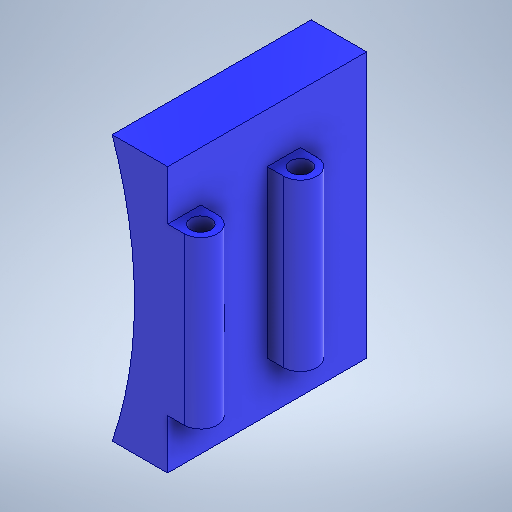
# Autodesk Inventor part: hand2_13
Saved by Autodesk Inventor 2025.1 (Build 291241000, 241)
## iProperties
Created: 2025-02-05
Part Number: hand2_13
Material: ABS プラスチック
Document SubType Name: Modeling
Designer: ryogo
Density: 1.06 g/cm^3
Appearance: 青 - 壁塗料 - 光沢
Author: ryogo
Autodesk Inventor part; units mm, degrees
ref_plane "YZ Plane" through (0, 0, 0) normal (1, 0, 0) x (0, 1, 0)
ref_plane "XZ Plane" through (0, 0, 0) normal (0, 1, 0) x (-1, 0, 0)
sketch "スケッチ1" plane through (0, 0, 0) normal (0, 1, 0) x (-1, 0, 0)
  line L0 (0, 0) -> (0, -30)
  circle A0 centre (0, 0) radius 3.05
  circle A1 centre (0, -30) radius 3.05
  circle A2 centre (0, 0) radius 5
  circle A3 centre (0, -30) radius 5
  line L1 (5, 0) -> (5, -30)
  line L2 (0, -5) -> (5, -5)
  line L3 (0, -25) -> (5, -25)
  line L4 (0, 5) -> (5, 5)
  line L5 (5, 5) -> (5, 0)
  line L6 (0, -35) -> (5, -35)
  line L7 (5, -35) -> (5, -30)
  line L8 (5, 5) -> (10, 5)
  line L9 (10, 5) -> (10, -35)
  line L10 (10, -35) -> (5, -35)
  line L11 (5, -35) -> (5, 5)
  dimension "d0" = 30
  dimension "d1" = 6.1
  dimension "d2" = 6.1
  dimension "d3" = 10
  dimension "d4" = 10
  dimension "d5" = 5
  dimension "d6" = 40
  constraints: 24 end point, 8 tangent, 7 point on circle, 4 centre point, 4 coincident, 4 point on line, 3 parallel, 2 horizontal, 2 perpendicular, 1 vertical
  measures "d0" distance of L0.start L0.end
  measures "d1" diameter of A0
  measures "d2" diameter of A1
  measures "d3" diameter of A2
  measures "d4" diameter of A3
  measures "d5" distance of L9.end L10.end
  measures "d6" distance between parallel lines of L8 L10
extrude "押し出し1" add sketch "スケッチ1" along normal blind 50 contours A2 | A2 L1 L2 | L3 L1 A3 | A3 | L4 L5 A2 | L5 L8 L9 L10 L7 L1 | L7 L6 A3
sketch "スケッチ2" plane through (0, 50, 0) normal (0, 1, 0) x (1, 0, 0)
  line L0 (-10, 35) -> (-10, -5) projected
  line L1 (0, 35) -> (-10, 35) projected
  line L2 (-10, -5) -> (-5, -5)
  line L3 (-5, -5) -> (-5, 35)
  line L4 (-5, 35) -> (-10, 35)
  line L5 (-10, 35) -> (-10, -5)
  point P0 (0, 0)
  constraints: 8 end point, 2 parallel, 1 horizontal, 1 midpoint, 1 perpendicular
extrude "押し出し2" add sketch "スケッチ2" along normal blind 15
sketch "スケッチ3" plane through (0, 0, 0) normal (0, -1, 0) x (1, 0, 0)
  line L0 (-10, 5) -> (0, 5) projected
  line L1 (-5, -35) -> (-5, -25) projected
  line L2 (-10, 5) -> (-5, 5)
  line L3 (-5, 5) -> (-5, -35)
  line L4 (-5, -35) -> (-10, -35)
  line L5 (-10, -35) -> (-10, 5)
  point P0 (0, 0)
  constraints: 8 end point, 2 parallel, 1 horizontal, 1 perpendicular
extrude "押し出し3" add sketch "スケッチ3" along normal blind 15
sketch "スケッチ4" plane through (-5, 0, -25) normal (1, 0, 0) x (0, 0, -1)
  circle A0 centre (-15, 25) radius 7
  line L0 (-30, 0) -> (-30, 50) projected
  line L1 (-20, 0) -> (-30, 0) projected
  point P0 (-25, 0)
  dimension "d13" = 14
  dimension "d14" = 15
  dimension "d15" = 25
  constraints: 1 centre point
  measures "d13" diameter of A0
  measures "d14" distance from line of A0.centre L0
  measures "d15" distance from line of L1 A0.centre
extrude "押し出し4" cut sketch "スケッチ4" along normal blind 50
sketch "スケッチ5" plane through (0, 0, -35) normal (0, 0, -1) x (-1, 0, 0)
  line L0 (10, -15) -> (10, 65) projected
  line L1 (10, 65) -> (5, 65) projected
  line L2 (10, -15) -> (5, -15)
  line L3 (5, -15) -> (5, 65)
  line L4 (5, 65) -> (10, 65)
  line L5 (10, 65) -> (10, -15)
  point P0 (0, 0)
  constraints: 8 end point, 2 parallel, 1 horizontal, 1 perpendicular
extrude "押し出し5" add sketch "スケッチ5" along normal blind 20
ref_plane "作業平面1" through (-10, -13, 5) normal (-1, 0, 0) x (0, 0, 1)
sketch "スケッチ6" plane through (-10, -13, 5) normal (-1, 0, 0) x (0, 0, 1)
  line L0 (0, -2) -> (0, 78) projected
  line L1 (0, 78) -> (-60, 78) projected
  line L2 (-60, -2) -> (-60, 78) projected
  line L3 (0, -2) -> (-60, -2) projected
  point P0 (-5, 13)
extrude "押し出し6" add sketch "スケッチ6" along normal blind 5
sketch "スケッチ7" plane through (-5, 0, 5) normal (0, 0, 1) x (1, 0, 0)
  line L0 (-10, 63) -> (-10, -13) projected
  line L1 (-10, 25) -> (-132.5, 25)
  circle A0 centre (-132.5, 25) radius 122.5
  line L2 (-10, 65) -> (-16.7146, 65)
  line L3 (0, -15) -> (-10, -15) projected
  line L4 (-10, -15) -> (-16.7146, -15)
  line L5 (0, 0) -> (5, 0) projected
  line L6 (5, 0) -> (5, 50) projected
  line L7 (0, 50) -> (5, 50) projected
  line L8 (0, 50) -> (0, 65) projected
  line L9 (0, 65) -> (-10, 65) projected
  line L10 (-10, -15) -> (-10, 65) projected
  line L11 (0, -15) -> (-10, -15) projected
  line L12 (0, 0) -> (0, -15) projected
  dimension "d23" = 122.5
  dimension "d24" = 180
  constraints: 6 end point, 3 point on circle, 2 horizontal, 1 centre point, 1 coincident, 1 midpoint
  measures "d23" distance of L1.start L1.end
  measures "d24" angle of L3 L4
extrude "押し出し7" add sketch "スケッチ7" against normal blind 60 contours L0 A0 L2 L10 | L0 L10 L4 A0
